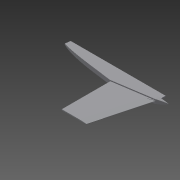
# Autodesk Inventor part: wing
Saved by Autodesk Inventor 2014 SP1 (Build 180222100, 222)
## iProperties
Created: 2018-05-06
Part Number: wing
Material: Generic
Document SubType Name: Modeling
Designer: Dadang
Density: 1 g/cm^3
Appearance: Default
Author: Dadang
Autodesk Inventor part; units mm, degrees
ref_plane "XZ Plane" through (0, 0, 0) normal (0, 1, 0) x (-1, 0, 0)
ref_plane "XY Plane" through (0, 0, 0) normal (0, 0, 1) x (1, 0, 0)
sketch "Sketch1" plane through (0, 0, 0) normal (0, 0, 1) x (1, 0, 0)
  line L0 (0, 0) -> (31.107, -13.144) construction
  line L1 (31.107, -13.144) -> (90.4342, -24.316) construction
  line L2 (90.4342, -24.316) -> (170, -35) construction
  spline S0 degree 3 poles (0, 0) (31.107, -13.144) (90.4342, -24.316) (170, -35) knots 1 1 1 1 2 2 2 2
  line L3 (0, 0) -> (0, 25)
  line L4 (0, 25) -> (458.1698, 25)
  line L5 (263.9103, -47.6101) -> (170, -35)
  line L6 (263.9103, -47.6101) -> (263.9103, -280)
  line L7 (263.9103, -280) -> (383.9103, -280)
  line L8 (458.1698, 25) -> (458.1698, 0)
  line L9 (458.1698, 0) -> (498.1698, 0)
  line L10 (453.2023, -18.73) -> (383.9103, -280)
  line L11 (498.1698, 0) -> (453.2023, -18.73)
  line L12 (263.9103, -47.6101) -> (453.2023, -18.73)
  line L13 (0, 0) -> (458.1698, 0)
  dimension "d5" = 25
  dimension "d21" = 120
  dimension "d22" = 40
  constraints: 22 end point, 3 perpendicular, 1 collinear, 3 other
  measures "d5" distance of L0.start L3.end
  measures "d21" distance of L6.end L7.end
  measures "d22" distance of L8.end L9.end
extrude "Extrusion1" add sketch "Sketch1" along normal blind 5
fillet "Fillet4" radius 2.5 2 edges at (263.9103, -163.8051, 5) (263.9103, -163.8051, 0)
chamfer "Chamfer3" distance 30 angle 4 1 edges at (418.5563, -149.365, 5) measured on face at (367.8409, -115.5586, 5)
chamfer "Chamfer4" distance 30 angle 4 1 edges at (418.5563, -149.365, 0) measured on face at (367.8409, -115.5586, 0)
extrude "Extrusion2" add sketch "Sketch1" along normal mid plane 20 contours L13 L9 L11 L12 L5 S0
ref_plane "Work Plane1" through (0, 0, 0) normal (1, 0, 0) x (0, 1, 0)
sketch "Sketch3" plane through (170, -35, 0) normal (-0.1330842, -0.9911047, 0) x (0.9911047, -0.1330842, 0)
  line L0 (94.7531, 5) -> (97.2755, 5) projected
  line L1 (-173.1458, 0) -> (-173.1458, 5) projected
  line L2 (-173.1458, 5) -> (-142.2369, 8.2112) construction
  line L3 (-142.2369, 8.2112) -> (-88.1915, 8.8084) construction
  line L4 (-88.1915, 8.8084) -> (-64.664, 9.327) construction
  line L5 (-64.664, 9.327) -> (-17.8895, 10) construction
  line L6 (-17.8895, 10) -> (0, 10) construction
  spline S0 degree 4 poles (-173.1458, 5) (-142.2369, 8.2112) (-88.1915, 8.8084) (-64.664, 9.327) (-17.8895, 10) (0, 10) knots 1 1 1 1 1 2 3 3 3 3 3
  line L7 (-173.1458, 0) -> (-142.2369, -5) construction
  line L8 (-142.2369, -5) -> (-106.8114, -6.5671) construction
  line L9 (-106.8114, -6.5671) -> (-87.8107, -8.4635) construction
  line L10 (-87.8107, -8.4635) -> (-64.664, -9.0617) construction
  line L11 (-64.664, -9.0617) -> (-17.6017, -10) construction
  line L12 (-17.6017, -10) -> (0, -10) construction
  spline S1 degree 4 poles (-173.1458, 0) (-142.2369, -5) (-106.8114, -6.5671) (-87.8107, -8.4635) (-64.664, -9.0617) (-17.6017, -10) (0, -10) knots 1 1 1 1 1 2 3 4 4 4 4 4
  line L13 (0, 10) -> (0, 26.8531)
  line L14 (0, 26.8531) -> (-182.9789, 26.8531)
  line L15 (-182.9789, 26.8531) -> (-182.9789, -21.0643)
  line L16 (-182.9789, -21.0643) -> (0, -21.0643)
  line L17 (0, -21.0643) -> (0, -10)
  constraints: 10 end point, 3 parallel, 3 perpendicular, 1 collinear, 6 other
extrude "Extrusion3" cut sketch "Sketch3" against normal blind 700
sketch "Sketch4" plane through (498.1698, 0, -10) normal (0.3845031, -0.9231237, 0) x (0.9231237, 0.3845031, 0)
  line L0 (-48.7123, 12.9022) -> (-86.5095, 15) projected
  line L1 (-86.5095, 10) -> (-48.7123, 12.0978) projected
  line L2 (0, 0) -> (-48.7123, 0) projected
  line L3 (0, 0) -> (0, 20) projected
  line L4 (-48.7123, 20) -> (0, 20) projected
  line L5 (-48.7123, 15) -> (-48.7123, 20) projected
  line L6 (-48.7123, 0) -> (-21.0795, 3.0362) construction
  line L7 (-21.0795, 3.0362) -> (-8.2996, 6.9919) construction
  line L8 (-8.2996, 6.9919) -> (0, 12.5) construction
  spline S0 degree 3 poles (-48.7123, 0) (-21.0795, 3.0362) (-8.2996, 6.9919) (0, 12.5) knots 1 1 1 1 2 2 2 2
  line L9 (-48.7123, 20) -> (-30.6011, 18.9948) construction
  line L10 (-30.6011, 18.9948) -> (-9.6534, 16.7372) construction
  line L11 (-9.6534, 16.7372) -> (0, 12.5) construction
  spline S1 degree 3 poles (-48.7123, 20) (-30.6011, 18.9948) (-9.6534, 16.7372) (0, 12.5) knots 1 1 1 1 2 2 2 2
  line L12 (-48.7123, 20) -> (-47.6447, 29.9058)
  line L13 (-47.6447, 29.9058) -> (10.2478, 29.9058)
  line L14 (10.2478, 29.9058) -> (12.4288, -9.391)
  line L15 (12.4288, -9.391) -> (-49.7244, -9.391)
  line L16 (-49.7244, -9.391) -> (-48.7123, 0)
  point P0 (-459.8723, 10)
  constraints: 10 end point, 3 parallel, 3 perpendicular, 1 point on line, 6 other
extrude "Extrusion4" cut sketch "Sketch4" against normal blind 700
body "Solid1"
